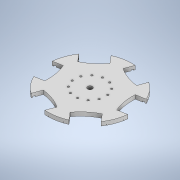
# Autodesk Inventor part: hub
Saved by Autodesk Inventor 2021 (Build 250183000, 183)
## iProperties
Created: 2022-10-17
Part Number: hub
Material: Generic
Document SubType Name: Modeling
Designer: Jonathan
Density: 1 g/cm^3
Appearance: Default
roller_angle: 40.00 deg
wheel_d: 6.000 in
roller_d: 1.000 in
roller_shaft_d: 0.125 in
roller_count: 6.000 ul
hub_d: 5.500 in
shaft_d: 0.315 in
hub_t: 0.250 in
roller_side_gap: 0.063 in
roller_back_gap: 0.063 in
roller_shaft_l: 2.000 in
Author: Jonathan
Autodesk Inventor part; units mm, degrees
ref_plane "YZ Plane" through (0, 0, 0) normal (1, 0, 0) x (0, 1, 0)
ref_plane "XZ Plane" through (0, 0, 0) normal (0, 1, 0) x (-1, 0, 0)
ref_plane "XY Plane" through (0, 0, 0) normal (0, 0, 1) x (1, 0, 0)
sketch "Sketch2" plane through (0, 0, 0) normal (0, 1, 0) x (-1, 0, 0)
  circle A0 centre (0, 0) radius 69.85
  circle A1 centre (0, 0) radius 4
  dimension "d10" = 139.7
  dimension "d36" = 8
  constraints: 2 centre point, 2 coincident
  measures "d10" diameter of A0
  measures "d36" diameter of A1
extrude "Extrusion1" add sketch "Sketch2" along normal blind 6.35
sketch "Sketch3" plane through (0, 0, 0) normal (0, 1, 0) x (-1, 0, 0)
  line L0 (-9.7351, -77.547) -> (0, -50.8) construction
  line L1 (0, -50.8) -> (-32.6536, -38.9151) construction
  line L2 (-32.6536, -38.9151) -> (-42.3887, -65.6621) construction
  line L3 (0, 0) -> (0, -50.8) construction
  line L4 (0, 0) -> (-32.6536, -38.9151) construction
  circle A0 centre (0, 0) radius 50.8 construction
  circle A1 centre (0, 0) radius 76.2 construction
  line L5 (-9.7351, -77.547) -> (-42.3887, -65.6621)
  line L6 (-1.0478, -53.6789) -> (-33.7014, -41.7939) construction
  line L7 (-9.7351, -77.547) -> (-1.0478, -53.6789) construction
  line L8 (-42.3887, -65.6621) -> (-33.7014, -41.7939) construction
  line L9 (-9.7351, -77.547) -> (-8.2434, -78.09)
  line L10 (-8.2434, -78.09) -> (0.1843, -54.9351)
  line L11 (-35.4528, -41.9643) -> (-43.8805, -65.1191)
  line L12 (-43.8805, -65.1191) -> (-42.3887, -65.6621)
  line L13 (-9.0486, -75.6608) -> (-41.7022, -63.7759) construction
  line L14 (-1.7343, -55.5651) -> (-34.388, -43.6801) construction
  line L15 (-26.0619, -71.6046) -> (-25.3754, -69.7184) construction
  line L16 (-18.0611, -49.6226) -> (-17.3746, -47.7364) construction
  arc A2 (-1.7343, -55.5651) -> (-34.388, -43.6801) centre (-43.4366, -119.341) ccw construction
  arc A3 (0.1843, -54.9351) -> (-35.4528, -41.9643) centre (-43.4366, -119.341) ccw
  line L17 (-17.3746, -47.7364) -> (-16.8317, -46.2446) construction
  dimension "d14" = 101.6
  dimension "d15" = 40
  dimension "d16" = 152.4
  dimension "d17" = 1.5875
  dimension "d24" = 1.5875
  constraints: 36 end point, 11 point on circle, 7 point on line, 5 perpendicular, 4 centre point, 4 equal length, 3 coincident, 3 collinear, 3 midpoint, 2 tangent, 1 parallel, 1 vertical
  measures "d14" diameter of A0
  measures "d15" angle of L4 L3
  measures "d16" diameter of A1
  measures "d17" distance between parallel lines of L2 L11
  measures "d24" distance of L16.end L17.end
extrude "Extrusion2" cut sketch "Sketch3" along normal blind 6.35
pattern_circular "Circular Pattern2" count 6 over 360 about axis through (0, -10, 0) along (0, 1, 0) of "Extrusion2"
sketch "Sketch4" plane through (0, 0, 0) normal (0, 1, 0) x (-1, 0, 0)
  circle A0 centre (0, 0) radius 76.2 construction
  circle A1 centre (0, 0) radius 50.8 construction
  line L0 (0, 0) -> (0, -50.8) construction
  line L1 (0, 0) -> (-32.6536, -38.9151) construction
  line L2 (0, -50.8) -> (-32.6536, -38.9151) construction
  line L3 (0, -50.8) -> (-9.7351, -77.547) construction
  line L4 (-9.7351, -77.547) -> (-42.3887, -65.6621) construction
  line L5 (-42.3887, -65.6621) -> (-32.6536, -38.9151) construction
  line L6 (-26.0619, -71.6046) -> (-21.7183, -59.6705) construction
  line L7 (-21.7183, -59.6705) -> (-17.3746, -47.7364) construction
  line L8 (2.6929, -66.866) -> (2.1499, -68.3578)
  line L9 (2.1499, -68.3578) -> (1.607, -69.8496)
  line L10 (1.607, -69.8496) -> (-46.1294, -52.4749)
  line L11 (-46.1294, -52.4749) -> (-45.5865, -50.9832)
  line L12 (-45.5865, -50.9832) -> (-45.0435, -49.4914)
  line L13 (-45.0435, -49.4914) -> (2.6929, -66.866)
  line L14 (2.1499, -68.3578) -> (-21.7183, -59.6705) construction
  line L15 (-21.7183, -59.6705) -> (-45.5865, -50.9832) construction
  dimension "d25" = 101.6
  dimension "d26" = 152.4
  dimension "d27" = 40
  dimension "d28" = 3.175
  dimension "d29" = 50.8
  constraints: 32 end point, 6 perpendicular, 4 collinear, 3 equal length, 3 point on circle, 3 point on line, 2 centre point, 2 coincident, 1 midpoint, 1 tangent, 1 vertical
  measures "d25" diameter of A1
  measures "d26" diameter of A0
  measures "d27" angle of L0 L1
  measures "d28" distance between parallel lines of L10 L13
  measures "d29" distance of L9.end L10.end
sketch "Sketch5" plane through (0, 0, 0) normal (0, 1, 0) x (-1, 0, 0)
  circle A0 centre (0, 0) radius 50.8 construction
  line L0 (0, 0) -> (0, -50.8) construction
  line L1 (0, 0) -> (-8.6873, -23.8682) construction
  line L2 (-8.6873, -23.8682) -> (-17.3746, -47.7364) construction
  circle A1 centre (-8.6873, -23.8682) radius 1.5875
  dimension "d37" = 101.6
  dimension "d39" = 20
  dimension "d40" = 3.175
  constraints: 6 end point, 2 centre point, 2 coincident, 2 collinear, 2 point on circle, 1 vertical
  measures "d37" diameter of A0
  measures "d39" angle of L0 L1
  measures "d40" diameter of A1
extrude "Extrusion3" cut sketch "Sketch5" along normal blind 6.35
pattern_circular "Circular Pattern4" count 12 over 360 about axis through (0, -10, 0) along (0, 1, 0) of "Extrusion3"
extrude "Extrusion4" cut sketch "Sketch4" along normal blind 1.5875
pattern_circular "Circular Pattern5" count 6 over 360 about axis through (0, -10, 0) along (0, 1, 0) of "Extrusion4"
equation "\"d10\" = hub_d"
equation "\"d36\" = shaft_d"
equation "\"d12\" = hub_t"
equation "\"d14\" = wheel_d - 2 * roller_d"
equation "\"d15\" = roller_angle"
equation "\"d16\" = wheel_d"
equation "\"d17\" = roller_side_gap"
equation "\"d24\" = roller_back_gap"
equation "\"d19\" = hub_t"
equation "\"d25\" = wheel_d - 2 * roller_d"
equation "\"d26\" = wheel_d"
equation "\"d27\" = roller_angle"
equation "\"d28\" = roller_shaft_d"
equation "\"d29\" = roller_shaft_l"
equation "\"d37\" = wheel_d - 2 * roller_d"
equation "\"d39\" = 0.5 * roller_angle"
equation "\"d40\" = hub_bolt_d"
equation "\"d41\" = hub_t"
equation "\"d46\" = 0.5 * roller_shaft_d"
equation "\"roller_angle\" = 40deg"
equation "\"wheel_d\" = 152.4"
equation "\"roller_d\" = 25.4"
equation "\"roller_shaft_d\" = 3.175"
equation "\"roller_count\" = 6"
equation "\"hub_d\" = 139.7"
equation "\"shaft_d\" = 8"
equation "\"hub_t\" = 6.35"
equation "\"roller_side_gap\" = 1.5875"
equation "\"roller_back_gap\" = 1.5875"
equation "\"roller_shaft_l\" = 50.8"
equation "\"hub_bolt_d\" = 3.175"
body "Solid1"
